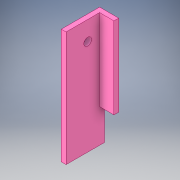
# Autodesk Inventor part: LiftAngleBracketExtensionRight
Saved by Autodesk Inventor 2017 SP1 (Build 210196100, 196)
## iProperties
Created: 2016-08-26
Part Number: LiftAngleBracketExtensionRight
Material: Aluminum 6061
Document SubType Name: Modeling
Designer: steele
Density: 2.7 g/cm^3
Appearance: Pink
Author: steele
Autodesk Inventor part; units mm, degrees
ref_plane "YZ Plane" through (0, 0, 0) normal (1, 0, 0) x (0, 1, 0)
ref_plane "XZ Plane" through (0, 0, 0) normal (0, 1, 0) x (-1, 0, 0)
ref_plane "XY Plane" through (0, 0, 0) normal (0, 0, 1) x (1, 0, 0)
sketch "Sketch1" plane through (0, 0, 0) normal (0, 1, 0) x (-1, 0, 0)
  line L0 (0, 0) -> (0, -50.8)
  line L1 (0, -50.8) -> (-50.8, -50.8)
  line L2 (-50.8, -50.8) -> (-50.8, -44.45)
  line L3 (-50.8, -44.45) -> (-6.35, -44.45)
  line L4 (-6.35, -44.45) -> (-6.35, 0)
  line L5 (-6.35, 0) -> (0, 0)
  dimension "d0" = 6.35
  dimension "d1" = 50.8
  constraints: 12 end point, 7 perpendicular, 1 vertical
  measures "d0" distance of L4.end L0.start
  measures "d1" distance of L0.end L1.end
extrude "Extrusion1" add sketch "Sketch1" along normal blind 152.4
sketch "Sketch4" plane through (6.35, 0, -44.45) normal (0, 0, 1) x (1, 0, 0)
  line L0 (44.45, 0) -> (0, 0) projected
  line L1 (0, 0) -> (0, 152.4) projected
  line L2 (44.45, 0) -> (0, 0)
  line L3 (0, 0) -> (0, 44.45)
  line L4 (0, 44.45) -> (44.45, 44.45)
  line L5 (44.45, 44.45) -> (44.45, 0)
  point P0 (-6.35, 0)
  dimension "d8" = 44.45
  constraints: 8 end point, 2 parallel, 1 horizontal, 1 perpendicular, 1 point on line
  measures "d8" distance of L4.end L0.start
extrude "Extrusion3" cut sketch "Sketch4" against normal through all
sketch "Sketch5" plane through (6.35, 152.4, -44.45) normal (0, 0, 1) x (1, 0, 0)
  line L0 (44.45, -107.95) -> (44.45, 0) projected
  line L1 (44.45, 0) -> (-6.35, 0) projected
  line L2 (44.45, -107.95) -> (19.05, -107.95)
  line L3 (19.05, -107.95) -> (19.05, 0)
  line L4 (19.05, 0) -> (44.45, 0)
  line L5 (44.45, 0) -> (44.45, -107.95)
  point P0 (-6.35, -152.4)
  dimension "d11" = 25.4
  constraints: 8 end point, 2 parallel, 1 horizontal, 1 midpoint, 1 perpendicular
  measures "d11" distance between parallel lines of L0 L3
extrude "Extrusion4" cut sketch "Sketch5" against normal through all
sketch "Sketch6" plane through (0, 0, -50.8) normal (-1, 0, 0) x (0, 0, 1)
  line L0 (0, 152.4) -> (50.8, 152.4) projected
  line L1 (0, 0) -> (0, 152.4) projected
  point P0 (50.8, 0)
  point P1 (22.225, 127)
  dimension "d14" = 25.4
  dimension "d15" = 22.225
  measures "d14" distance from line of point (22.225, 127) L0
  measures "d15" distance from line of point (22.225, 127) L1
hole "Hole1" at (0, 127, -28.575) direction (1, 0, 0) diameter 10.0838 end through all clearance for "Flat Head Machine Screw (82)" size "3/8" standard "Ansi Unified Screw Threads"
body "Solid1"
